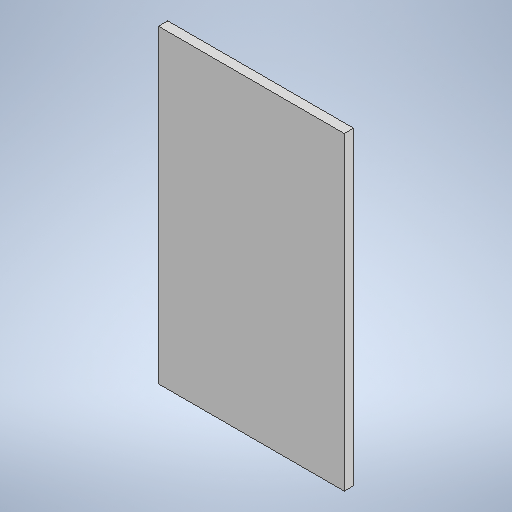
# Autodesk Inventor part: AcrylicPane
Saved by Autodesk Inventor 2025.1 (Build 291241020, 241B)
## iProperties
Created: 2024-09-25
Part Number: AcrylicPane
Material: Generic
Document SubType Name: Modeling
Designer: Si Teng Wu
Density: 1 g/cm^3
Appearance: Default
Author: Si Teng Wu
Autodesk Inventor part; units mm, degrees
ref_plane "YZ Plane" through (0, 0, 0) normal (1, 0, 0) x (0, 1, 0)
ref_plane "XZ Plane" through (0, 0, 0) normal (0, 1, 0) x (-1, 0, 0)
ref_plane "XY Plane" through (0, 0, 0) normal (0, 0, 1) x (1, 0, 0)
sketch "Sketch1" plane through (0, 0, 0) normal (0, 0, 1) x (1, 0, 0)
  line L0 (-30, 50) -> (30, 50)
  line L1 (30, 50) -> (30, -50)
  line L2 (30, -50) -> (-30, -50)
  line L3 (-30, -50) -> (-30, 50)
  point P0 (0, 0)
  point P1 (0, 50)
  dimension "d0" = 50
  dimension "d2" = 100
  dimension "d3" = 60
  dimension "d4" = 30
  constraints: 8 end point, 2 parallel, 1 horizontal, 1 midpoint, 1 perpendicular
  measures "d0" distance of point (0, 50) point (0, 0)
  measures "d2" distance between parallel lines of L2 L0
  measures "d3" distance between parallel lines of L1 L3
  measures "d4" distance from line of L3 point (0, 0)
extrude "Extrusion1" add sketch "Sketch1" along normal blind 3
body "Solid1"
